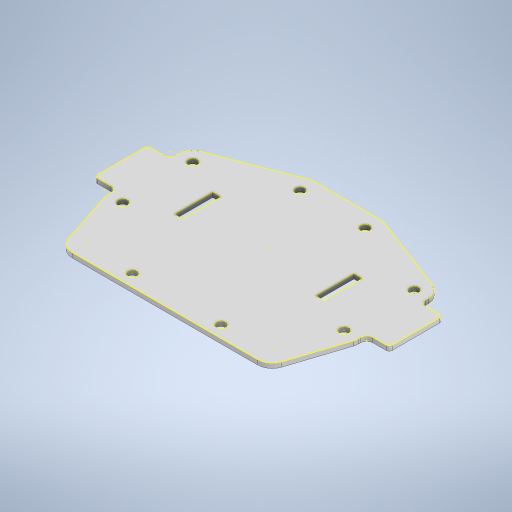
# Autodesk Inventor part: plytka_glowna
Saved by Autodesk Inventor 2023 (Build 270158000, 158)
## iProperties
Created: 2024-04-24
Part Number: plytka_glowna
Material: Ogólny
Document SubType Name: Modeling
Designer: Kamil
Density: 1 g/cm^3
Appearance: Domyślna
Author: Kamil
Autodesk Inventor part; units mm, degrees
ref_plane "YZ Plane" through (0, 0, 0) normal (1, 0, 0) x (0, 1, 0)
ref_plane "XZ Plane" through (0, 0, 0) normal (0, 1, 0) x (-1, 0, 0)
ref_plane "XY Plane" through (0, 0, 0) normal (0, 0, 1) x (1, 0, 0)
sketch "Szkic1" plane through (0, 0, 0) normal (0, 1, 0) x (-1, 0, 0)
  circle A0 centre (-37.45, -11.85) radius 1.6
  circle A1 centre (-11, -21.7) radius 1.55
  circle A2 centre (-15, 31) radius 1.6
  line L0 (-25.3, 6.4859) -> (-22.5, 6.4859)
  line L1 (-22.5, 6.4859) -> (-22.5, -6.4859)
  line L2 (-22.5, -6.4859) -> (-25.3, -6.4859)
  line L3 (-25.3, -6.4859) -> (-25.3, 6.4859)
  line L4 (-42.3, 11.85) -> (-42.3, 11)
  arc A3 (-44.3, 9) -> (-42.3, 11) centre (-44.3, 11) ccw
  line L5 (-44.3, 9) -> (-49.9, 9)
  line L6 (-49.9, 9) -> (-49.9, -9)
  line L7 (-49.9, -9) -> (-44.3, -9)
  arc A4 (-42.3, -11) -> (-44.3, -9) centre (-44.3, -11) ccw
  line L8 (-42.3, -11) -> (-42.3, -11.85)
  arc A5 (-42.3, -11.85) -> (-39.0298, -16.4355) centre (-37.45, -11.85) ccw
  line L9 (-12, -26.7) -> (12, -26.7)
  line L10 (35, 35) -> (-35, 35)
  line L11 (0, -26.7) -> (0, 35)
  line L12 (-49.9, 0) -> (-32, 0)
  circle A6 centre (-37.45, 11.85) radius 1.6
  arc A7 (-42.0609, 13.3541) -> (-42.3, 11.85) centre (-37.45, 11.85) ccw
  line L13 (-35, 35) -> (-42.0609, 13.3541)
  line L14 (-12, -26.7) -> (-39.1714, -16.3842)
  arc A8 (42.3, 11) -> (44.3, 9) centre (44.3, 11) ccw
  line L15 (25.3, 6.4859) -> (22.5, 6.4859)
  line L16 (44.3, 9) -> (49.9, 9)
  line L17 (22.5, 6.4859) -> (22.5, -6.4859)
  line L18 (25.3, -6.4859) -> (25.3, 6.4859)
  line L19 (49.9, 9) -> (49.9, -9)
  line L20 (22.5, -6.4859) -> (25.3, -6.4859)
  line L21 (49.9, -9) -> (44.3, -9)
  arc A9 (44.3, -9) -> (42.3, -11) centre (44.3, -11) ccw
  line L22 (42.3, -11) -> (42.3, -11.85)
  circle A10 centre (37.45, -11.85) radius 1.6
  arc A11 (39.0298, -16.4355) -> (42.3, -11.85) centre (37.45, -11.85) ccw
  circle A12 centre (11, -21.7) radius 1.55
  line L23 (42.3, 11.85) -> (42.3, 11)
  circle A13 centre (15, 31) radius 1.6
  line L24 (49.9, 0) -> (32, 0)
  circle A14 centre (37.45, 11.85) radius 1.6
  arc A15 (42.3, 11.85) -> (42.0609, 13.3541) centre (37.45, 11.85) ccw
  line L25 (35, 35) -> (42.0609, 13.3541)
  line L26 (12, -26.7) -> (39.1714, -16.3842)
  point P0 (0, 0)
  point P1 (-22.5, 0)
  point P2 (-39.0298, 16.4355)
  point P3 (22.5, 0)
  point P4 (39.0298, 16.4355)
  dimension "d5" = 12.9718
  dimension "d6" = 2.8
  dimension "d8" = 22.5
  dimension "d9" = 24
  dimension "d12" = 24.6
  dimension "d13" = 5.6
  dimension "d14" = 5.6
  dimension "d17" = 2.85
  dimension "d18" = 20.2141
  dimension "d19" = 35
  constraints: 56 end point, 30 symmetric about line, 18 point on circle, 16 centre point, 5 perpendicular, 4 horizontal, 4 midpoint, 3 vertical, 2 tangent, 1 horizontal alignment, 1 vertical alignment, 15 other
  measures "d5" distance of L0.end L1.end
  measures "d6" distance of L0.start L0.end
  measures "d8" distance from line of L1 point (0, 0)
  measures "d9" distance of L9.start L9.end
  measures "d12" distance between parallel lines of L6 L3
  measures "d13" distance of L5.start L5.end
  measures "d14" distance of L6.end L7.end
  measures "d17" vertical distance of L6.end A0.centre
  measures "d18" distance between parallel lines of L2 L9
  measures "d19" distance of L10.end L11.end
extrude "Wyciągnięcie proste1" add sketch "Szkic1" along normal blind 1.6
fillet "Zaokrąglenie1" radius 5 2 edges at (-35, 0.8, 35) (35, 0.8, 35)
fillet "Zaokrąglenie3" radius 1 4 edges at (-49.9, 0.8, -9) (-49.9, 0.8, 9) (49.9, 0.8, 9) (49.9, 0.8, -9)
sketch "Szkic4" plane through (0, 1.6, 0) normal (0, 1, 0) x (1, 0, 0)
  arc A0 (49.9, 8) -> (48.9, 9) centre (48.9, 8) ccw projected
  line L0 (48.9, 9) -> (44.3, 9) projected
  arc A1 (42.3, 11) -> (44.3, 9) centre (44.3, 11) ccw projected
  line L1 (42.3, 11) -> (42.3, 11.85) projected
  arc A2 (42.3, 11.85) -> (39.1714, 16.3842) centre (37.45, 11.85) ccw projected
  line L2 (39.1714, 16.3842) -> (12, 26.7) projected
  line L3 (12, 26.7) -> (-12, 26.7) projected
  line L4 (-12, 26.7) -> (-39.1714, 16.3842) projected
  arc A3 (-39.1714, 16.3842) -> (-42.3, 11.85) centre (-37.45, 11.85) ccw projected
  line L5 (-42.3, 11.85) -> (-42.3, 11) projected
  arc A4 (-44.3, 9) -> (-42.3, 11) centre (-44.3, 11) ccw projected
  line L6 (-44.3, 9) -> (-48.9, 9) projected
  arc A5 (-48.9, 9) -> (-49.9, 8) centre (-48.9, 8) ccw projected
  line L7 (-49.9, 8) -> (-49.9, -8) projected
  arc A6 (-49.9, -8) -> (-48.9, -9) centre (-48.9, -8) ccw projected
  line L8 (-48.9, -9) -> (-44.3, -9) projected
  arc A7 (-42.3, -11) -> (-44.3, -9) centre (-44.3, -11) ccw projected
  line L9 (-42.3, -11) -> (-42.3, -11.85) projected
  arc A8 (-42.3, -11.85) -> (-42.0609, -13.3541) centre (-37.45, -11.85) ccw projected
  line L10 (-42.0609, -13.3541) -> (-36.1252, -31.5506) projected
  arc A9 (-36.1252, -31.5506) -> (-31.3717, -35) centre (-31.3717, -30) ccw projected
  line L11 (-31.3717, -35) -> (31.3717, -35) projected
  arc A10 (31.3717, -35) -> (36.1252, -31.5506) centre (31.3717, -30) ccw projected
  line L12 (36.1252, -31.5506) -> (42.0609, -13.3541) projected
  arc A11 (42.0609, -13.3541) -> (42.3, -11.85) centre (37.45, -11.85) ccw projected
  line L13 (42.3, -11.85) -> (42.3, -11) projected
  arc A12 (44.3, -9) -> (42.3, -11) centre (44.3, -11) ccw projected
  line L14 (44.3, -9) -> (48.9, -9) projected
  arc A13 (48.9, -9) -> (49.9, -8) centre (48.9, -8) ccw projected
  line L15 (49.9, -8) -> (49.9, 8) projected
  line L16 (25.3, -6.4859) -> (22.5, -6.4859) projected
  line L17 (22.5, -6.4859) -> (22.5, 6.4859) projected
  line L18 (22.5, 6.4859) -> (25.3, 6.4859) projected
  line L19 (25.3, 6.4859) -> (25.3, -6.4859) projected
  circle A14 centre (37.45, 11.85) radius 1.6 projected
  circle A15 centre (11, 21.7) radius 1.55 projected
  circle A16 centre (37.45, -11.85) radius 1.6 projected
  circle A17 centre (15, -31) radius 1.6 projected
  circle A18 centre (-15, -31) radius 1.6 projected
  circle A19 centre (-37.45, 11.85) radius 1.6 projected
  circle A20 centre (-37.45, -11.85) radius 1.6 projected
  circle A21 centre (-11, 21.7) radius 1.55 projected
  line L20 (-25.3, -6.4859) -> (-25.3, 6.4859) projected
  line L21 (-25.3, 6.4859) -> (-22.5, 6.4859) projected
  line L22 (-22.5, 6.4859) -> (-22.5, -6.4859) projected
  line L23 (-22.5, -6.4859) -> (-25.3, -6.4859) projected
  point P0 (0, 0)
